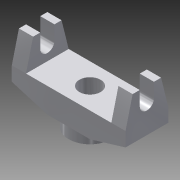
# Autodesk Inventor part: 5.3
Saved by Autodesk Inventor 2015 SP2 (Build 190223200, 223)
## iProperties
Created: 2015-09-23
Part Number: 5.3
Material: Aluminum 6061
Document SubType Name: Modeling
Designer: KC-019
Density: 2.7 g/cm^3
Appearance: Aluminum - Flat
Author: KC-019
Autodesk Inventor part; units mm, degrees
ref_plane "YZ Plane" through (0, 0, 0) normal (1, 0, 0) x (0, 1, 0)
ref_plane "XZ Plane" through (0, 0, 0) normal (0, 1, 0) x (-1, 0, 0)
ref_plane "XY Plane" through (0, 0, 0) normal (0, 0, 1) x (1, 0, 0)
sketch "Sketch1" plane through (0, 0, 0) normal (0, 0, 1) x (1, 0, 0)
  line L0 (0, 0) -> (203.2, 0)
  line L1 (203.2, 0) -> (203.2, 95.25)
  line L2 (203.2, 95.25) -> (0, 95.25)
  line L3 (0, 95.25) -> (0, 0)
  dimension "d0" = 95.25
  dimension "d1" = 203.2
  constraints: 8 end point, 2 parallel, 1 horizontal, 1 perpendicular
  measures "d0" distance of L2.end L0.start
  measures "d1" distance of L0.start L0.end
extrude "Extrusion1" add sketch "Sketch1" along normal blind 76.2
sketch "Sketch2" plane through (0, 0, 76.2) normal (0, 0, 1) x (1, 0, 0)
  line L0 (0, 95.25) -> (0, 19.05)
  line L1 (0, 95.25) -> (0, 0) projected
  line L2 (0, 0) -> (203.2, 0) projected
  line L3 (101.6, 0) -> (63.5, 0)
  line L4 (63.5, 0) -> (139.7, 0)
  line L5 (63.5, 0) -> (0, 19.05)
  line L6 (203.2, 95.25) -> (203.2, 19.05)
  line L7 (203.2, 0) -> (203.2, 95.25) projected
  line L8 (203.2, 19.05) -> (139.7, 0)
  line L9 (0, 19.05) -> (0, 0)
  line L10 (203.2, 19.05) -> (203.2, 0)
  dimension "d4" = 76.2
  dimension "d5" = 38.1
  dimension "d6" = 76.2
  dimension "d7" = 76.2
  constraints: 16 end point, 4 point on line, 2 collinear, 1 midpoint
  measures "d4" distance of L0.start L0.end
  measures "d5" distance of L3.start L3.end
  measures "d6" distance of L3.end L4.end
  measures "d7" distance of L6.start L6.end
extrude "Extrusion2" cut sketch "Sketch2" against normal blind 76.2
sketch "Sketch3" plane through (0, 0, 76.2) normal (0, 0, 1) x (1, 0, 0)
  line L0 (0, 19.05) -> (0, 44.45)
  line L1 (0, 95.25) -> (0, 19.05) projected
  line L2 (203.2, 19.05) -> (203.2, 44.45)
  line L3 (203.2, 19.05) -> (203.2, 95.25) projected
  line L4 (0, 95.25) -> (25.4, 95.25)
  line L5 (203.2, 95.25) -> (0, 95.25) projected
  line L6 (25.4, 95.25) -> (25.4, 44.45)
  line L7 (203.2, 95.25) -> (177.8, 95.25)
  line L8 (177.8, 95.25) -> (177.8, 44.45)
  line L9 (177.8, 44.45) -> (25.4, 44.45)
  point P0 (0, 0)
  dimension "d10" = 25.4
  dimension "d11" = 25.4
  dimension "d12" = 25.4
  dimension "d13" = 25.4
  constraints: 14 end point, 4 point on line, 3 perpendicular
  measures "d10" distance of L0.start L0.end
  measures "d11" distance of L2.start L2.end
  measures "d12" distance of L1.start L4.end
  measures "d13" distance of L3.end L7.end
extrude "Extrusion3" cut sketch "Sketch3" against normal blind 76.2
sketch "Sketch4" plane through (0, 95.25, 0) normal (-1, 0, 0) x (0, 0, 1)
  line L0 (76.2, 0) -> (76.2, -50.8)
  line L1 (63.5, 0) -> (76.2, 0)
  line L2 (0, 0) -> (12.7, 0)
  line L3 (63.5, 0) -> (76.2, 0)
  line L4 (63.5, 0) -> (76.2, -50.8)
  line L5 (76.2, -50.8) -> (76.2, 0)
  line L6 (76.2, 0) -> (63.5, 0)
  line L7 (12.7, 0) -> (0, 0)
  line L8 (76.2, -50.8) -> (63.5, 0)
  line L9 (76.2, 0) -> (76.2, -50.8)
  line L10 (0, -50.8) -> (0, 0)
  line L11 (0, -50.8) -> (0, 0) projected
  line L12 (0, -50.8) -> (12.7, 0)
  point P0 (0, -95.25)
  point P1 (0, -76.2)
  point P2 (76.2, -76.2)
  dimension "d17" = 50.8
  dimension "d20" = 12.7
  dimension "d21" = 12.7
  dimension "d22" = 50.8
  constraints: 24 end point, 5 collinear
  measures "d17" distance of L2.end L1.start
  measures "d20" distance of L2.start L2.end
  measures "d21" distance of L1.start L0.start
  measures "d22" distance of L0.start L0.end
extrude "Extrusion4" cut sketch "Sketch4" against normal through all
sketch "Sketch6" plane through (0, 19.05, 0) normal (-1, 0, 0) x (0, 0, 1)
  line L0 (63.5, 76.2) -> (12.7, 76.2) projected
  arc A0 (25.4, 50.8) -> (50.8, 50.8) centre (38.1, 50.8) ccw
  line L1 (25.4, 50.8) -> (25.4, 76.2)
  line L2 (50.8, 50.8) -> (50.8, 76.2)
  line L3 (25.4, 76.2) -> (50.8, 76.2)
  point P0 (0, -19.05)
  dimension "d28" = 25.4
  constraints: 6 end point, 2 perpendicular, 2 point on circle, 2 point on line, 2 tangent, 1 centre point, 1 collinear
  measures "d28" diameter of A0
extrude "Extrusion5" cut sketch "Sketch6" against normal through all
sketch "Sketch7" plane through (63.5, 0, 0) normal (0, -1, 0) x (1, 0, 0)
  line L0 (0, 76.2) -> (0, 0) projected
  line L1 (76.2, 0) -> (76.2, 76.2) projected
  line L2 (0, 76.2) -> (76.2, 76.2) projected
  line L3 (0, 0) -> (76.2, 0) projected
  circle A0 centre (38.1, 38.1) radius 38.1
  point P0 (-63.5, 0)
  constraints: 1 centre point
extrude "Extrusion6" add sketch "Sketch7" along normal blind 19.05 contours A0
sketch "Sketch9" plane through (25.4, 44.45, 76.2) normal (0, 1, 0) x (1, 0, 0)
  arc A0 (76.2, 0) -> (114.3, 38.1) centre (76.2, 38.1) ccw projected
  circle A1 centre (76.2, 38.1) radius 19.05
  point P0 (-25.4, 76.2)
  dimension "d33" = 38.1
  constraints: 1 centre point, 1 coincident
  measures "d33" diameter of A1
extrude "Extrusion7" cut sketch "Sketch9" along normal blind 63.5
sketch "Sketch11" plane through (101.6, -19.05, 38.1) normal (0, -1, 0) x (1, 0, 0)
  circle A0 centre (0, 0) radius 19.05
  point P0 (-101.6, -38.1)
  dimension "d36" = 38.1
  constraints: 1 centre point
  measures "d36" diameter of A0
extrude "Extrusion8" cut sketch "Sketch11" against normal blind 63.5
body "Solid1"
